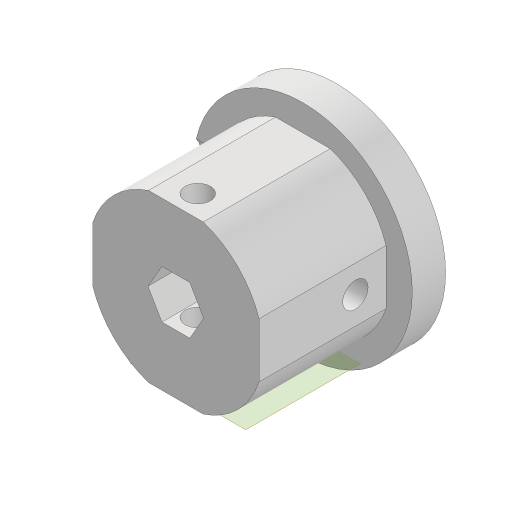
# Autodesk Inventor part: 3mm_shaft_couple_sideclip_v3
Saved by Autodesk Inventor 2023 (Build 270158000, 158)
## iProperties
Created: 2020-09-24
Part Number: 3mm_shaft_couple_sideclip_v3
Material: Generic
Document SubType Name: Modeling
Designer: CDT
Density: 1 g/cm^3
Appearance: Default
Author: CDT
Autodesk Inventor part; units mm, degrees
ref_plane "YZ Plane" through (0, 0, 0) normal (1, 0, 0) x (0, 1, 0)
ref_plane "XZ Plane" through (0, 0, 0) normal (0, 1, 0) x (-1, 0, 0)
ref_plane "XY Plane" through (0, 0, 0) normal (0, 0, 1) x (1, 0, 0)
sketch "Sketch1" plane through (0, 0, 0) normal (0, 0, 1) x (1, 0, 0)
  circle A0 centre (0, 0) radius 10
  dimension "d0" = 20
  constraints: 1 centre point, 1 coincident
  measures "d0" diameter of A0
extrude "Extrusion1" add sketch "Sketch1" along normal blind 14.5
sketch "Sketch2" plane through (0, 0, 0) normal (0, 0, -1) x (-1, 0, 0)
  line L0 (-1.5, -2.5) -> (1.5, -2.5)
  line L1 (1.5, -2.5) -> (1.5, 2.5)
  line L2 (1.5, 2.5) -> (-1.5, 2.5)
  line L3 (-1.5, 2.5) -> (-1.5, -2.5)
  point P0 (0, 0)
  dimension "d3" = 3
  dimension "d4" = 5
  dimension "d5" = 2.5
  dimension "d6" = 1.5
  constraints: 8 end point, 2 parallel, 1 horizontal, 1 perpendicular
  measures "d3" distance of L2.end L1.end
  measures "d4" distance of L1.end L0.end
  measures "d5" distance from line of L2 point (0, 0)
  measures "d6" distance from line of L3 point (0, 0)
extrude "Extrusion2" cut sketch "Sketch2" against normal blind 10
sketch "Sketch4" plane through (0, 0, 0) normal (0, 0, -1) x (-1, 0, 0)
  circle A0 centre (0, 0) radius 4.5
  dimension "d12" = 9
  constraints: 1 centre point, 1 coincident
  measures "d12" diameter of A0
extrude "Extrusion4" [suppressed]
sketch "Sketch10" plane through (0, 0, 14.5) normal (0, 0, 1) x (1, 0, 0)
  line L0 (1.59, 2.754) -> (3.18, 0)
  line L1 (3.18, 0) -> (1.59, -2.754)
  line L2 (1.59, -2.754) -> (-1.59, -2.754)
  line L3 (-1.59, -2.754) -> (-3.18, 0)
  line L4 (-3.18, 0) -> (-1.59, 2.754)
  line L5 (-1.59, 2.754) -> (1.59, 2.754)
  point P0 (0, 0)
  point P1 (0, 0)
  dimension "d63" = 3.18
  constraints: 12 end point, 1 coincident, 13 other
  measures "d63" distance of L4.end L0.start
extrude "Extrusion7" cut sketch "Sketch10" against normal blind 9
ref_plane "Work Plane3" through (0, -10, 0) normal (0, -1, 0) x (1, 0, 0)
sketch "Sketch11" plane through (0, -10, 0) normal (0, -1, 0) x (1, 0, 0)
  circle A0 centre (0, 12) radius 1.45
  line L0 (10, 14.5) -> (-10, 14.5) projected
  point P0 (0, 0)
  dimension "d66" = 2.9
  dimension "d128" = 2.5
  constraints: 1 centre point
  measures "d66" diameter of A0
  measures "d128" distance from line of L0 A0.centre
extrude "Extrusion8" cut sketch "Sketch11" against normal through all
ref_plane "Work Plane4" through (-10.5, -2.5, 0) normal (-1, 0, 0) x (0, 0, 1)
sketch "Sketch12" plane through (-10.5, -2.5, 0) normal (-1, 0, 0) x (0, 0, 1)
  circle A0 centre (3.5, 2.5) radius 1.45
  line L0 (0, 0) -> (5.5, 0) projected
  point P0 (0, 2.5)
  dimension "d71" = 2.9
  dimension "d74" = 3.5
  dimension "d124" = 2.5
  constraints: 1 centre point
  measures "d71" diameter of A0
  measures "d74" distance of point (0, 2.5) A0.centre
  measures "d124" distance from line of L0 A0.centre
extrude "Extrusion9" cut sketch "Sketch12" against normal blind 22
sketch "Sketch16" plane through (0, 0, 0) normal (0, 0, -1) x (-1, 0, 0)
  line L0 (-13.5, 7.2115) -> (-9.5, 7.2115)
  line L1 (-9.5, 7.2115) -> (-9.5, -8.6118)
  line L2 (-9.5, -8.6118) -> (-13.5, -8.6118)
  line L3 (-13.5, -8.6118) -> (-13.5, 7.2115)
  line L4 (9.5, 9.312) -> (14.5, 9.312)
  line L5 (14.5, 9.312) -> (14.5, -11.179)
  line L6 (14.5, -11.179) -> (9.5, -11.179)
  line L7 (9.5, -11.179) -> (9.5, 9.312)
  line L8 (-14.4464, 13.5) -> (12.1592, 13.5)
  line L9 (12.1592, 13.5) -> (12.1592, 9.5)
  line L10 (12.1592, 9.5) -> (-14.4464, 9.5)
  line L11 (-14.4464, 9.5) -> (-14.4464, 13.5)
  line L12 (-12.7193, -13.5) -> (12.1592, -13.5)
  line L13 (12.1592, -13.5) -> (12.1592, -9.5)
  line L14 (12.1592, -9.5) -> (-12.7193, -9.5)
  line L15 (-12.7193, -9.5) -> (-12.7193, -13.5)
  line L16 (1.5, -2.5) -> (-1.5, -2.5) projected
  line L17 (-1.5, -2.5) -> (-1.5, 2.5) projected
  line L18 (-1.5, 2.5) -> (1.5, 2.5) projected
  line L19 (1.5, 2.5) -> (1.5, -2.5) projected
  point P0 (-12.5, -8.5)
  point P1 (11.5, -8.5)
  point P2 (11.5, 8.5)
  point P3 (8.5, 8.5)
  point P4 (9.5, -9.5)
  point P5 (-8.5, -8.5)
  point P6 (12.1592, 9.312)
  point P7 (12.1592, -11.179)
  dimension "d104" = 4
  dimension "d105" = 7
  dimension "d106" = 8
  dimension "d107" = 7
  dimension "d108" = 8
  dimension "d109" = 5
  dimension "d110" = 4
  dimension "d111" = 4
  constraints: 32 end point, 8 parallel, 4 horizontal, 4 perpendicular, 1 point on line
  measures "d104" distance between parallel lines of L12 L14
  measures "d105" distance between parallel lines of L16 L14
  measures "d106" distance between parallel lines of L1 L17
  measures "d107" distance between parallel lines of L10 L18
  measures "d108" distance between parallel lines of L7 L19
  measures "d109" distance between parallel lines of L5 L7
  measures "d110" distance between parallel lines of L3 L1
  measures "d111" distance between parallel lines of L8 L10
extrude "Extrusion13" cut sketch "Sketch16" against normal through all contours L0 L1 L2 L3 | L4 L5 L6 L13 L14 L7 | L14 L13 L6 L7 | L7 L6 L13 L12 L15 L14 | L8 L9 L10 L11
sketch "Sketch18" plane through (0, 0, 0) normal (0, 0, -1) x (-1, 0, 0)
  circle A0 centre (0, 0) radius 12.5
  line L0 (-1.5, -2.5) -> (-1.5, 2.5) projected
  line L1 (1.5, 2.5) -> (1.5, -2.5) projected
  line L2 (-1.5, 2.5) -> (1.5, 2.5)
  line L3 (1.5, 2.5) -> (1.5, -2.5)
  line L4 (1.5, -2.5) -> (-1.5, -2.5)
  line L5 (-1.5, -2.5) -> (-1.5, 2.5)
  dimension "d118" = 25
  constraints: 8 end point, 2 parallel, 1 centre point, 1 coincident, 1 horizontal, 1 perpendicular
  measures "d118" diameter of A0
extrude "Extrusion15" add sketch "Sketch18" along normal blind 3.8
chamfer "Chamfer1" distance 4.75 angle 45 4 edges at (1.5, 0, -3.8) (0, 2.5, -3.8) (0, -2.5, -3.8) (-1.5, 0, -3.8)
sketch "Sketch19" plane through (-9.5, -3.1225, 14.5) normal (-1, 0, 0) x (0, 0, 1)
  circle A0 centre (-11, 3.1225) radius 1.45 projected
  circle A1 centre (-11, 3.1225) radius 4.5
  point P0 (-14.5, 3.1225)
  dimension "d125" = 9
  constraints: 1 centre point, 1 coincident
  measures "d125" diameter of A1
extrude "Extrusion16" cut sketch "Sketch19" along normal blind 5 contours A0 | A1
equation "\"d5\" = 0.5 * d4"
equation "\"d6\" = 0.5 * d3"
equation "\"d107\" = d105"
equation "\"d108\" = d106"
body "Solid1"
